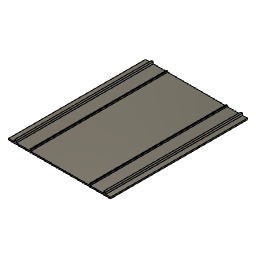
Animation v5 (Autodesk Fusion 360 archive; units mm, degrees)
design "Floor"
Autodesk Fusion 360 part; units mm, degrees
sketch "Sketch1" plane through (0, 0, 0) normal (0, 1, 0) x (1, 0, 0)
  line L0 (0, 0) -> (-140, 0)
  line L1 (-140, 0) -> (-140, 140)
  line L2 (-140, 140) -> (0, 140)
  line L3 (0, 140) -> (0, 0)
  dimension "d1" = 140
  dimension "d2" = 140
  constraint horizontal L0
  constraint vertical L1
  constraint horizontal L2
  constraint vertical L3
  constraint coincident L0.start L3.end
  measures "d1" distance of L0.start L0.end
  measures "d2" distance of L0.start L2.end
extrude "Extrude1" add sketch "Sketch1" along normal blind 2 makes body 1
sketch "Sketch2" plane through (0, 2, 0) normal (0, 1, 0) x (-1, 0, 0)
  line L0 (0, -140) -> (140, -140)
  line L1 (140, -140) -> (140, 0)
  line L2 (140, 0) -> (0, 0)
  line L3 (0, 0) -> (0, -140)
  line L4 (70, -140) -> (23, -140)
  line L5 (117, -140) -> (116, -140)
  line L6 (117, -140) -> (117.75, -140)
  line L7 (117.75, -140) -> (116.25, -140)
  line L8 (117.75, -140) -> (116.25, -140)
  line L9 (116.25, -140) -> (116.25, 0)
  line L10 (116.25, 0) -> (117.75, 0)
  line L11 (117.75, 0) -> (117.75, -140)
  dimension "d5" = 47
  dimension "d6" = 47
  dimension "d7" = 0.75
  dimension "d8" = 1.5
  constraint midpoint L0 L4.start
  constraint parallel L0 L4
  constraint parallel L0 L6
  constraint horizontal L7
  constraint horizontal L8
  constraint vertical L9
  constraint horizontal L10
  constraint vertical L11
  constraint coincident L2 L9.end
  measures "d5" distance of L4.start L5.start
  measures "d6" distance of L4.start L4.end
  measures "d7" distance of L5.start L6.end
  measures "d8" distance of L6.end L7.end
extrude "Extrude2" add sketch "Sketch2" along normal blind 2 contours L0 L2 L5 L6 L7 L8 L9 L10 L11 bodies 1
sketch "Sketch3" plane through (0, 2, 0) normal (0, 1, 0) x (-1, 0, 0)
  line L0 (116.25, -140) -> (116.25, 0)
  line L1 (116.25, 0) -> (0, 0)
  line L2 (0, 0) -> (0, -140)
  line L3 (0, -140) -> (116.25, -140)
  line L4 (0, -140) -> (22.25, -140)
  line L5 (22.25, -140) -> (20.75, -140)
  line L6 (20.75, -140) -> (20.75, 0)
  line L7 (20.75, 0) -> (22.25, 0)
  line L8 (22.25, 0) -> (22.25, -140)
  dimension "d11" = 22.25
  dimension "d12" = 1.5
  constraint coincident L2.end L3.start
  constraint perpendicular L2 L4
  constraint horizontal L5
  constraint vertical L6
  constraint horizontal L7
  constraint vertical L8
  measures "d11" distance of L2.end L4.end
  measures "d12" distance of L4.end L5.end
extrude "Extrude3" add sketch "Sketch3" along normal blind 2 contours L1 L3 L4 L5 L6 L7 L8 bodies 1
sketch "Sketch4" plane through (0, 2, 0) normal (0, 1, 0) x (-1, 0, 0)
extrude "Extrude4" add 1 faces at (0, 0.6667, -93.3333) along direction (1, 0, 0) blind 10 on bodies 1 bodies 1
extrude "Extrude5" add 1 faces at (-140, 0.6667, -46.6667) along direction (-1, 0, 0) blind 10 on bodies 1 bodies 1
sketch "Sketch5" plane through (0, 2, 0) normal (0, 1, 0) x (-1, 0, 0)
  line L0 (20.75, -140) -> (20.75, 0)
  line L1 (20.75, 0) -> (-10, 0)
  line L2 (-10, 0) -> (-10, -140)
  line L3 (-10, -140) -> (20.75, -140)
  line L4 (0.75, -140) -> (-2.25, -140)
  line L5 (-2.25, -140) -> (-2.25, 0)
  line L6 (-2.25, 0) -> (0.75, 0)
  line L7 (0.75, 0) -> (0.75, -140)
  dimension "d19" = 20
  dimension "d20" = 3
  dimension "d21" = 140
  constraint horizontal L4
  constraint vertical L5
  constraint horizontal L6
  constraint vertical L7
  measures "d19" distance of L0.start L4.start
  measures "d20" distance of L4.start L4.end
  measures "d21" distance of L4.start L6.end
extrude "Extrude6" add sketch "Sketch5" along normal blind 3 contours L1 L3 L4 L5 L6 L7 bodies 1
sketch "Sketch6" plane through (0, 2, 0) normal (0, 1, 0) x (-1, 0, 0)
  line L0 (117.75, 0) -> (117.75, -140)
  line L1 (117.75, -140) -> (150, -140)
  line L2 (150, -140) -> (150, 0)
  line L3 (150, 0) -> (117.75, 0)
  line L4 (137.75, -140) -> (140.75, -140)
  line L5 (140.75, -140) -> (140.75, 0)
  line L6 (140.75, 0) -> (137.75, 0)
  line L7 (137.75, 0) -> (137.75, -140)
  dimension "d24" = 20
  dimension "d25" = 3
  dimension "d26" = 140
  constraint horizontal L4
  constraint vertical L5
  constraint horizontal L6
  constraint vertical L7
  measures "d24" distance of L0.end L4.start
  measures "d25" distance of L4.start L4.end
  measures "d26" distance of L4.start L6.end
extrude "Extrude7" add sketch "Sketch6" along normal blind 3 contours L1 L3 L4 L5 L6 L7 bodies 1
sketch "Sketch7" plane through (0, 5, 0) normal (0, 1, 0) x (-1, 0, 0)
sketch "Sketch8" plane through (0, 2, 0) normal (0, 1, 0) x (-1, 0, 0)
sketch "Sketch9" plane through (0, 5, 0) normal (0, 1, 0) x (-1, 0, 0)
sketch "Sketch10" plane through (0, 5, 0) normal (0, 1, 0) x (-1, 0, 0)
sketch "Sketch11" plane through (0, 2, 0) normal (0, 1, 0) x (-1, 0, 0)
  line L0 (22.25, -140) -> (116.25, -140)
  line L1 (116.25, -140) -> (116.25, 0)
  line L2 (116.25, 0) -> (22.25, 0)
  line L3 (23.25, 0) -> (21.75, 0)
  line L4 (21.75, 0) -> (21.75, -140)
  line L5 (21.75, -140) -> (23.25, -140)
  line L6 (23.25, -140) -> (23.25, 0)
  dimension "d29" = 1
  dimension "d30" = 1.5
  constraint horizontal L3
  constraint vertical L4
  constraint horizontal L5
  constraint vertical L6
  measures "d29" distance of L2.end L3.start
  measures "d30" distance of L3.start L3.end
extrude "Extrude8" cut 1 faces at (-21.75, 4, -93.3333) along direction (0, -1, 0) blind 2 on bodies 1 bodies 1
extrude "Extrude9" add sketch "Sketch11" along normal blind 2 contours L0 L2 L3 L4 L5 L6 bodies 1
extrude "Extrude10" cut 1 faces at (-116.75, 4, -93.3333) along direction (0, -1, 0) blind 2 on bodies 1 bodies 1
sketch "Sketch12" plane through (0, 2, 0) normal (0, 1, 0) x (-1, 0, 0)
  line L0 (23.25, 0) -> (23.25, -140)
  line L1 (23.25, -140) -> (137.75, -140)
  line L2 (137.75, -140) -> (137.75, 0)
  line L3 (137.75, 0) -> (23.25, 0)
  line L4 (23.25, -140) -> (115.25, -140)
  line L5 (115.25, -140) -> (116.75, -140)
  line L6 (116.75, -140) -> (116.75, 0)
  line L7 (116.75, 0) -> (115.25, 0)
  line L8 (115.25, 0) -> (115.25, -140)
  dimension "d37" = 92
  dimension "d38" = 1.5
  constraint coincident L0.end L1.start
  constraint perpendicular L0 L4
  constraint horizontal L5
  constraint vertical L6
  constraint horizontal L7
  constraint vertical L8
  measures "d37" distance of L0.end L4.end
  measures "d38" distance of L4.end L5.end
extrude "Extrude11" add sketch "Sketch12" along normal blind 2 contours L1 L3 L5 L6 L7 L8 bodies 1
sketch "Sketch13" plane through (0, 2, 0) normal (0, 1, 0) x (-1, 0, 0)
copy_body "Body->Comp1" bodies 1 removing the originals makes body 2 in component "Component"
extrude "Extrude1'" add 1 faces at (-92.5833, 0.6667, 0) along direction (0, 0, 1) blind 75 on bodies 2 bodies 2 in component "Component"
component "Component" placed x (1, 0, 0) y (0, 1, 0) z (0, 0, 1) at (0, 0, 0)
